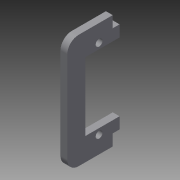
# Autodesk Inventor part: Servo Mount 080113
Saved by Autodesk Inventor 2013 (Build 170138000, 138)
## iProperties
Created: 2013-08-02
Part Number: Servo Mount 080113
Material: Generic
Document SubType Name: Modeling
Designer: Eric
Density: 1 g/cm^3
Author: Eric
Autodesk Inventor part; units mm, degrees
ref_plane "YZ Plane" through (0, 0, 0) normal (1, 0, 0) x (0, 1, 0)
ref_plane "XZ Plane" through (0, 0, 0) normal (0, 1, 0) x (-1, 0, 0)
ref_plane "XY Plane" through (0, 0, 0) normal (0, 0, 1) x (1, 0, 0)
sketch "Sketch1" plane through (0, 0, 0) normal (1, 0, 0) x (0, 1, 0)
  line L0 (30, 0) -> (35, 0)
  line L1 (35, 0) -> (35, 3)
  line L2 (35, 3) -> (40, 3)
  line L3 (40, 3) -> (40, 18)
  line L4 (35, 23) -> (-5, 23)
  line L5 (-10, 18) -> (-10, 3)
  line L6 (-10, 3) -> (-5, 3)
  line L7 (-5, 3) -> (-5, 0)
  line L8 (-5, 0) -> (0, 0)
  line L9 (0, 0) -> (0, 15)
  line L10 (0, 15) -> (30, 15)
  line L11 (30, 15) -> (30, 0)
  arc A0 (-5, 23) -> (-10, 18) centre (-5, 18) ccw
  arc A1 (40, 18) -> (35, 23) centre (35, 18) ccw
  point P0 (-10, 23)
  dimension "d0" = 5
  dimension "d1" = 3
  dimension "d2" = 5
  dimension "d3" = 20
  dimension "d4" = 30
  dimension "d5" = 12
  dimension "d6" = 5
  dimension "d7" = 3
  dimension "d8" = 5
  dimension "d9" = 5
  constraints: 24 end point, 4 point on circle, 4 tangent, 2 centre point, 2 perpendicular, 2 point on line, 1 equal radius, 1 parallel
  measures "d0" distance of L7.end L8.end
  measures "d1" distance of L6.end L7.end
  measures "d2" distance of L5.end L6.end
  measures "d3" distance of point (-10, 23) L5.end
  measures "d4" distance between parallel lines of L11 L9
  measures "d5" distance between parallel lines of L10 L6
  measures "d6" distance of L0.start L0.end
  measures "d7" distance of L0.end L1.end
  measures "d8" distance of L1.end L2.end
  measures "d9" radius of A0
extrude "Extrusion1" add sketch "Sketch1" along normal blind 3
sketch "Sketch3" plane through (3, 0, 0) normal (1, 0, 0) x (0, 0, -1)
  line L0 (0, 0) -> (-15, 0) projected
  line L1 (-15, 0) -> (-15, 30) projected
  line L2 (-15, 30) -> (0, 30) projected
  circle A0 centre (-9, 32.5) radius 1.5
  circle A1 centre (-9, -2.5) radius 1.5
  dimension "d12" = 3
  dimension "d14" = 3
  dimension "d15" = 6
  dimension "d16" = 6
  dimension "d17" = 2.5
  dimension "d18" = 2.5
  constraints: 2 centre point
  measures "d12" diameter of A0
  measures "d14" diameter of A1
  measures "d15" distance from line of L1 A1.centre
  measures "d16" distance from line of L1 A0.centre
  measures "d17" distance from line of L2 A0.centre
  measures "d18" distance from line of A1.centre L0
extrude "Extrusion2" cut sketch "Sketch3" against normal blind 3
body "Solid1"
